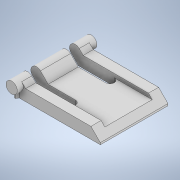
# Autodesk Inventor part: Part1
Saved by Autodesk Inventor 2020.2 (Build 242310000, 310)
## iProperties
Created: 2020-03-21
Part Number: Part1
Material: Generic
Document SubType Name: Modeling
Designer: daniel.gerdes
Density: 1 g/cm^3
Appearance: Default
Author: daniel.gerdes
Autodesk Inventor part; units mm, degrees
ref_plane "YZ Plane" through (0, 0, 0) normal (1, 0, 0) x (0, 1, 0)
ref_plane "XZ Plane" through (0, 0, 0) normal (0, 1, 0) x (-1, 0, 0)
ref_plane "XY Plane" through (0, 0, 0) normal (0, 0, 1) x (1, 0, 0)
sketch "Sketch3" plane through (0, 0, 0) normal (0, 1, 0) x (-1, 0, 0)
  line L0 (11.3, 9) -> (-11.3, 9)
  line L1 (-11.3, 9) -> (-11.3, -9)
  line L2 (-11.3, -9) -> (11.3, -9)
  line L3 (11.3, -9) -> (11.3, 9)
  line L4 (11.3, 9) -> (-11.3, -9) construction
  line L5 (-11.3, 9) -> (11.3, -9) construction
  line L6 (11.3, 5.15) -> (0.3, 5.15) construction
  line L7 (11.3, 6.3) -> (0.3, 6.3)
  line L8 (0.3, 4) -> (11.3, 4)
  arc A0 (11.3, 4) -> (11.3, 6.3) centre (11.3, 5.15) ccw
  arc A1 (0.3, 6.3) -> (0.3, 4) centre (0.3, 5.15) ccw
  line L9 (11.3, -5.15) -> (0.3, -5.15) construction
  line L10 (11.3, -4) -> (0.3, -4)
  line L11 (0.3, -6.3) -> (11.3, -6.3)
  arc A2 (11.3, -6.3) -> (11.3, -4) centre (11.3, -5.15) ccw
  arc A3 (0.3, -4) -> (0.3, -6.3) centre (0.3, -5.15) ccw
  point P0 (0, 0)
  point P1 (5.8, 5.15)
  point P2 (5.8, -5.15)
  dimension "d4" = 18
  dimension "d5" = 22.6
  dimension "d6" = 11
  dimension "d7" = 11
  dimension "d8" = 2.3
  dimension "d9" = 2.3
  dimension "d10" = 12.6
  dimension "d11" = 6.3
  constraints: 28 end point, 8 point on circle, 8 tangent, 4 centre point, 4 midpoint, 4 parallel, 3 perpendicular, 2 point on line, 1 horizontal
  measures "d4" distance between parallel lines of L2 L0
  measures "d5" distance of L0.start L0.end
  measures "d6" distance from line of L3 L6.end
  measures "d7" distance from line of L9.end L3
  measures "d8" distance between parallel lines of L8 L7
  measures "d9" distance between parallel lines of L11 L10
  measures "d10" distance between parallel lines of L11 L7
  measures "d11" distance from line of point (0, 0) L7
extrude "Extrusion3" add sketch "Sketch3" along normal blind 3 contours L3 L7 A1 L8 L10 A3 L11 L2 L1 L0
sketch "Sketch4" plane through (-11.3, 0, -4) normal (-1, 0, 0) x (0, 0, 1)
  line L0 (-2.3, 3) -> (0, 3) projected
  line L1 (10.3, 0) -> (10.3, 3) projected
  line L2 (-2.3, 3) -> (10.3, 3)
  line L3 (10.3, 3) -> (10.3, 2)
  line L4 (10.3, 2) -> (-2.3, 2)
  line L5 (-2.3, 2) -> (-2.3, 3)
  point P0 (4, 0)
  dimension "d14" = 1
  constraints: 8 end point, 2 parallel, 1 horizontal, 1 perpendicular, 1 point on line
  measures "d14" distance between parallel lines of L4 L2
extrude "Extrusion4" cut sketch "Sketch4" against normal blind 30
chamfer "Chamfer1" distance 2.5 angle 45 1 edges at (11.3, 3, -7.65)
sketch "Sketch5" plane through (0, 0, 0) normal (0, 0, 1) x (1, 0, 0)
  circle A0 centre (-10.7, 3) radius 1.5
  line L0 (11.3, 0) -> (11.3, 0.5) projected
  line L1 (-11.7607, 1.9393) -> (-9.8213, 0)
  line L2 (-11.3, 0) -> (11.3, 0) projected
  line L3 (-9.6393, 4.0607) -> (-7.5787, 2)
  line L4 (-0.3, 2) -> (-11.3, 2) projected
  line L5 (-7.5787, 2) -> (-9.8213, 0)
  point P0 (0, 0)
  point P1 (-9.582, 2)
  dimension "d20" = 3
  dimension "d21" = 3
  dimension "d22" = 22
  dimension "d23" = 135
  dimension "d24" = 135
  constraints: 6 end point, 2 point on circle, 2 point on line, 2 tangent, 1 centre point
  measures "d20" diameter of A0
  measures "d21" vertical distance of A0.centre point (0, 0)
  measures "d22" distance from line of A0.centre L0
  measures "d23" angle of L3 L4
  measures "d24" angle of L2 L1
extrude "Extrusion5" add sketch "Sketch5" along normal mid plane 18
sketch "Sketch6" plane through (-11.7607, 1.9393, 9) normal (-0.7071, -0.7071, 0) x (-0.7071, 0.7071, 0)
  line L0 (6.2129, 16.9) -> (-25.5876, 16.9)
  line L1 (-25.5876, 16.9) -> (-25.5876, 1.1)
  line L2 (-25.5876, 1.1) -> (6.2129, 1.1)
  line L3 (6.2129, 1.1) -> (6.2129, 16.9)
  line L4 (6.2129, 16.9) -> (-25.5876, 1.1) construction
  line L5 (-25.5876, 16.9) -> (6.2129, 1.1) construction
  point P0 (-9.6874, 9)
  dimension "d27" = 15.8
  constraints: 12 end point, 2 midpoint, 2 parallel, 1 horizontal, 1 perpendicular
  measures "d27" distance of L2.end L0.start
extrude "Extrusion6" cut sketch "Sketch6" along normal blind 10
extrude "Extrusion7" add sketch "Sketch5" along normal mid plane 21.2 contours A0
sketch "Sketch7" plane through (0, 0, 0) normal (0, -1, 0) x (1, 0, 0)
  line L0 (-11.3, -9) -> (-11.7607, -9) projected
  line L1 (-11.3, -9) -> (-10.9536, -9.6)
  line L2 (-10.9536, -9.6) -> (-10.6536, -9.6)
  line L3 (-10.6536, -9.6) -> (-10.3072, -9)
  line L4 (-9.2, -9) -> (-11.7607, -9) projected
  point P0 (0, 0)
  point P1 (-9.6393, -9)
  dimension "d32" = 9.6
  dimension "d33" = 60
  dimension "d34" = 60
  dimension "d35" = 0.3
  constraints: 6 end point, 1 parallel, 1 point on line
  measures "d32" vertical distance of L2.end point (0, 0)
  measures "d33" angle of L3 L1
  measures "d34" angle of L4 L1
  measures "d35" distance of L1.end L2.end
extrude "Extrusion8" add sketch "Sketch7" against normal up to next
mirror "Mirror1" about plane through (0, 0, 0) normal (0, 0, 1) of "Extrusion8"
sketch "Sketch8" plane through (0, 0, 0) normal (0, -1, 0) x (1, 0, 0)
  line L0 (-9.8213, -6.3) -> (-0.3, -6.3) projected
  line L1 (-0.3, -6.3) -> (-24.4848, -6.3)
  line L2 (-24.4848, -6.3) -> (-24.4848, -4)
  line L3 (-24.4848, -4) -> (-0.3, -4)
  line L4 (-0.3, -4) -> (-0.3, -6.3)
  line L5 (-0.3, 4) -> (-7.5787, 4) projected
  line L6 (-0.3, 4) -> (-23.0411, 4)
  line L7 (-23.0411, 4) -> (-23.0411, 6.3)
  line L8 (-23.0411, 6.3) -> (-0.3, 6.3)
  line L9 (-0.3, 6.3) -> (-0.3, 4)
  line L10 (-0.3, -4) -> (-9.8213, -4) projected
  line L11 (-0.3, 6.3) -> (-9.8213, 6.3) projected
  point P0 (0, 0)
  constraints: 16 end point, 4 parallel, 2 collinear, 2 horizontal, 2 perpendicular
extrude "Extrusion9" cut sketch "Sketch8" against normal blind 10
equation "\"d7\" = d6"
equation "\"d9\" = d8"
equation "\"d11\" = 0.5 * d10"
body "Solid3"
